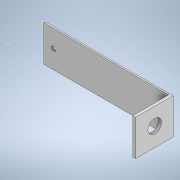
# Autodesk Inventor part: clamp 2 pipe
Saved by Autodesk Inventor 2020 (Build 240168000, 168)
## iProperties
Created: 2020-02-18
Part Number: clamp 2 pipe
Material: Generic
Document SubType Name: Modeling
Designer: Hp
Density: 1 g/cm^3
Appearance: Default
Author: Hp
Autodesk Inventor part; units mm, degrees
ref_plane "YZ Plane" through (0, 0, 0) normal (1, 0, 0) x (0, 1, 0)
ref_plane "XZ Plane" through (0, 0, 0) normal (0, 1, 0) x (-1, 0, 0)
ref_plane "XY Plane" through (0, 0, 0) normal (0, 0, 1) x (1, 0, 0)
sketch "Sketch1" plane through (0, 0, 0) normal (1, 0, 0) x (0, 1, 0)
  line L0 (1.8986, 1.3831) -> (-40.1014, 1.3831)
  line L1 (-40.1014, 1.3831) -> (-40.1014, -42.3731)
  line L2 (-40.1014, -42.3731) -> (1.8986, -42.3731)
  line L3 (1.8986, -42.3731) -> (1.8986, 1.3831)
  point P0 (0, 0)
  dimension "d0" = 42
  constraints: 8 end point, 2 parallel, 1 horizontal, 1 perpendicular
  measures "d0" distance of L2.end L1.end
extrude "Extrusion1" add sketch "Sketch1" along normal blind 100
sketch "Sketch3" plane through (0, 0, 0) normal (-1, 0, 0) x (0, 0, 1)
  point P0 (0, 0)
sketch "Sketch8" plane through (0, 0, 0) normal (-1, 0, 0) x (0, 0, 1)
  point P0 (0, 0)
  point P1 (-20.6894, -17.7504)
hole "Hole4" at (0, -17.7504, -20.6894) direction (1, 0, 0) diameter 15.875 end through all
sketch "Sketch9" plane through (0, -40.1014, 1.3831) normal (0, 0, 1) x (1, 0, 0)
  line L0 (0, 42) -> (100, 42) projected
  line L1 (0, 0) -> (100, 0) projected
  line L2 (1.351, 42) -> (99.1356, 42)
  line L3 (99.1356, 42) -> (99.1356, 0)
  line L4 (99.1356, 0) -> (1.351, 0)
  line L5 (1.351, 0) -> (1.351, 42)
  point P0 (0, 40.1014)
  point P1 (1.351, 0)
  constraints: 8 end point, 2 parallel, 2 point on line, 1 horizontal, 1 perpendicular
extrude "Extrusion4" cut sketch "Sketch9" against normal blind 42
sketch "Sketch10" plane through (1.351, -40.1014, 1.3831) normal (1, 0, 0) x (0, 0, -1)
  line L0 (0, 42) -> (42, 42) projected
  line L1 (43.7562, 0) -> (43.7562, 42) projected
  line L2 (0, 42) -> (43.7562, 42)
  line L3 (43.7562, 42) -> (43.7562, 0)
  line L4 (43.7562, 0) -> (0, 0)
  line L5 (0, 0) -> (0, 42)
  point P0 (1.3831, 40.1014)
  constraints: 8 end point, 2 parallel, 1 horizontal, 1 perpendicular
extrude "Extrusion5" cut sketch "Sketch10" against normal blind 25.4
sketch "Sketch11" plane through (0, -40.1014, -40.6169) normal (0, 0, 1) x (1, 0, 0)
  point P0 (0, 40.1014)
  point P1 (12.91, 21.6985)
hole "Hole5" at (12.91, -18.403, -40.6169) direction (0, 0, -1) diameter 5 end through all
sketch "Sketch12" plane through (100, 0, 0) normal (1, 0, 0) x (0, 0, -1)
  line L0 (42.3731, 1.8986) -> (-1.3831, 1.8986) projected
  line L1 (-1.3831, 1.8986) -> (42.3731, 1.8986)
  line L2 (42.3731, 1.8986) -> (42.3731, -40.1014)
  line L3 (42.3731, -40.1014) -> (-1.3831, -40.1014)
  line L4 (-1.3831, -40.1014) -> (-1.3831, 1.8986)
  point P0 (0, 0)
  constraints: 8 end point, 2 parallel, 1 horizontal, 1 perpendicular
extrude "Extrusion6" add sketch "Sketch12" along normal blind 50.8
sketch "Sketch13" plane through (99.1356, -40.1014, 1.3831) normal (-1, 0, 0) x (0, 0, 1)
  line L0 (-42, 42) -> (0, 42) projected
  line L1 (0, 42) -> (0, 0) projected
  line L2 (-42, 42) -> (0, 42)
  line L3 (0, 42) -> (0, 0)
  line L4 (0, 0) -> (-42, 0)
  line L5 (-42, 0) -> (-42, 42)
  point P0 (-1.3831, 40.1014)
  constraints: 8 end point, 2 parallel, 1 horizontal, 1 perpendicular
sketch "Sketch14" plane through (100, -17.7504, -20.6894) normal (-1, 0, 0) x (0, 0, 1)
  point P0 (20.6894, 17.7504)
  point P1 (-0.1562, -0.422)
hole "Hole6" at (100, -18.1724, -20.8455) direction (1, 0, 0) diameter 15.875 end through all
extrude "Extrusion7" cut sketch "Sketch13" against normal blind 48.26
sketch "Sketch15" plane through (0, -40.1014, -40.6169) normal (0, 0, 1) x (1, 0, 0)
  point P0 (0, 40.1014)
body "Solid1"
